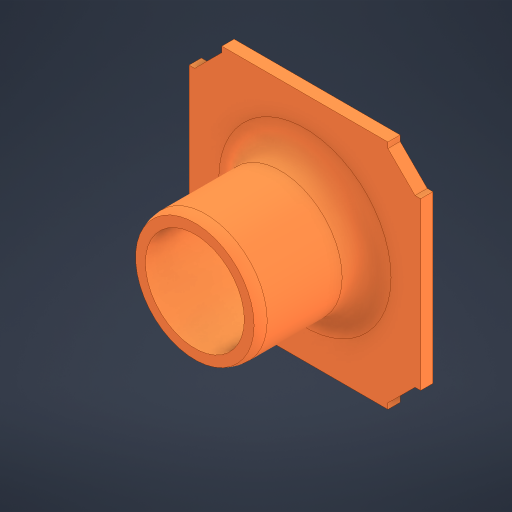
# Autodesk Inventor part: Objective Mount
Saved by Autodesk Inventor 2023.4 (Build 274418000, 418)
## iProperties
Created: 2022-08-09
Part Number: Objective Mount
Material: Generic
Document SubType Name: Modeling
Designer: xSibe
Density: 1 g/cm^3
Appearance: Plastic Orange
Author: xSibe
Autodesk Inventor part; units mm, degrees
ref_plane "YZ Plane" through (0, 0, 0) normal (1, 0, 0) x (0, 1, 0)
ref_plane "XZ Plane" through (0, 0, 0) normal (0, 1, 0) x (-1, 0, 0)
ref_plane "XY Plane" through (0, 0, 0) normal (0, 0, 1) x (1, 0, 0)
sketch "Sketch1" plane through (0, 0, 0) normal (0, 0, 1) x (1, 0, 0)
  circle A0 centre (-10, 20.9) radius 1.875 projected
  circle A1 centre (-10, -20.9) radius 1.875 projected
  circle A2 centre (10, 20.9) radius 1.875 projected
  circle A3 centre (10, -20.9) radius 1.875 projected
  circle A4 centre (20.8, -14.4) radius 2.075 projected
  circle A5 centre (20.8, 14.4) radius 2.075 projected
  circle A6 centre (-20.8, 14.4) radius 2.075 projected
  circle A7 centre (-20.8, -14.4) radius 2.075 projected
  line L0 (16.9, -16.9) -> (-16.9, -16.9) projected
  line L1 (-16.9, -16.9) -> (-16.9, 16.9) projected
  line L2 (-16.9, 16.9) -> (16.9, 16.9) projected
  line L3 (16.9, 16.9) -> (16.9, -16.9) projected
  line L4 (-17.05, 24.9) -> (-17.05, 22.55) projected
  line L5 (-17.05, 22.55) -> (-22.55, 17.05) projected
  line L6 (-22.55, 17.05) -> (-24.9, 17.05) projected
  line L7 (-24.9, 17.05) -> (-24.9, -17.05) projected
  line L8 (-24.9, -17.05) -> (-22.55, -17.05) projected
  line L9 (-22.55, -17.05) -> (-17.05, -22.55) projected
  line L10 (-17.05, -22.55) -> (-17.05, -24.9) projected
  line L11 (-17.05, -24.9) -> (17.05, -24.9) projected
  line L12 (17.05, -24.9) -> (17.05, -22.55) projected
  line L13 (17.05, -22.55) -> (22.55, -17.05) projected
  line L14 (22.55, -17.05) -> (24.9, -17.05) projected
  line L15 (24.9, -17.05) -> (24.9, 17.05) projected
  line L16 (24.9, 17.05) -> (22.55, 17.05) projected
  line L17 (22.55, 17.05) -> (17.05, 22.55) projected
  line L18 (17.05, 22.55) -> (17.05, 24.9) projected
  line L19 (17.05, 24.9) -> (-17.05, 24.9) projected
  line L20 (24.825, 16.975) -> (24.825, -16.975)
  line L21 (24.825, -16.975) -> (22.5189, -16.975)
  line L22 (22.5189, -16.975) -> (16.975, -22.5189)
  line L23 (16.975, -22.5189) -> (16.975, -24.825)
  line L24 (16.975, -24.825) -> (-16.975, -24.825)
  line L25 (-16.975, -24.825) -> (-16.975, -22.5189)
  line L26 (-16.975, -22.5189) -> (-22.5189, -16.975)
  line L27 (-22.5189, -16.975) -> (-24.825, -16.975)
  line L28 (-24.825, -16.975) -> (-24.825, 16.975)
  line L29 (-24.825, 16.975) -> (-22.5189, 16.975)
  line L30 (-22.5189, 16.975) -> (-16.975, 22.5189)
  line L31 (-16.975, 22.5189) -> (-16.975, 24.825)
  line L32 (-16.975, 24.825) -> (16.975, 24.825)
  line L33 (16.975, 24.825) -> (16.975, 22.5189)
  line L34 (16.975, 22.5189) -> (22.5189, 16.975)
  line L35 (22.5189, 16.975) -> (24.825, 16.975)
  line L36 (-24.825, 16.975) -> (-23.672, 16.975)
  line L37 (-23.672, 16.975) -> (-23.672, -16.975)
  line L38 (-23.672, -16.975) -> (-24.825, -16.975)
  line L39 (-24.825, -16.975) -> (-24.825, 16.975)
  line L40 (-16.975, 24.825) -> (16.975, 24.825)
  line L41 (16.975, 24.825) -> (16.975, 23.672)
  line L42 (16.975, 23.672) -> (-16.975, 23.672)
  line L43 (-16.975, 23.672) -> (-16.975, 24.825)
  line L44 (24.825, 16.975) -> (23.672, 16.975)
  line L45 (23.672, 16.975) -> (23.672, -16.975)
  line L46 (23.672, -16.975) -> (24.825, -16.975)
  line L47 (24.825, -16.975) -> (24.825, 16.975)
  line L48 (-16.975, -24.825) -> (16.975, -24.825)
  line L49 (16.975, -24.825) -> (16.975, -23.672)
  line L50 (16.975, -23.672) -> (-16.975, -23.672)
  line L51 (-16.975, -23.672) -> (-16.975, -24.825)
  point P0 (0, 0)
  dimension "d0" = 0.075
  constraints: 64 end point, 8 parallel, 4 horizontal, 4 midpoint, 4 perpendicular, 15 other
  measures "d0" distance between parallel lines of L15 L20
ref_plane "Work Plane1" through (-24.9, -24.9, 7.7) normal (0, 0, 1) x (1, 0, 0)
extrude "Extrusion1" add sketch "Sketch1" along normal blind 2.5 from surface at 7.7 contours A0 | A1 | A2 | A3 | A4 | A5 | A6 | A7 | L0 L1 L2 L3 | L45 L21 L22 L23 L50 L25 L26 L27 L37 L29 L30 L31 L42 L33 L34 L35
sketch "Sketch2" plane through (0, 0, 0) normal (0, 0, 1) x (1, 0, 0)
  line L0 (22.5189, 16.975) -> (23.672, 16.975) projected
  line L1 (16.975, 22.5189) -> (22.5189, 16.975) projected
  line L2 (16.975, 23.672) -> (16.975, 22.5189) projected
  line L3 (-16.975, 22.5189) -> (-16.975, 23.672) projected
  line L4 (-22.5189, 16.975) -> (-16.975, 22.5189) projected
  line L5 (-23.672, 16.975) -> (-22.5189, 16.975) projected
  line L6 (-22.5189, -16.975) -> (-23.672, -16.975) projected
  line L7 (-16.975, -22.5189) -> (-22.5189, -16.975) projected
  line L8 (-16.975, -23.672) -> (-16.975, -22.5189) projected
  line L9 (16.975, -22.5189) -> (16.975, -23.672) projected
  line L10 (22.5189, -16.975) -> (16.975, -22.5189) projected
  line L11 (23.672, -16.975) -> (22.5189, -16.975) projected
  line L12 (24.825, -16.975) -> (24.825, -24.825)
  line L13 (24.825, -24.825) -> (16.975, -24.825)
  line L14 (24.825, -24.825) -> (14.825, -24.825)
  line L15 (14.825, -24.825) -> (14.825, -19.825)
  line L16 (19.825, -14.825) -> (24.825, -14.825)
  line L17 (24.825, -14.825) -> (24.825, -24.825)
  line L18 (19.825, -14.825) -> (14.825, -19.825)
  line L19 (24.825, 24.825) -> (24.825, 14.825)
  line L20 (14.825, 24.825) -> (24.825, 24.825)
  line L21 (14.825, 19.825) -> (14.825, 24.825)
  line L22 (14.825, 19.825) -> (19.825, 14.825)
  line L23 (24.825, 14.825) -> (19.825, 14.825)
  line L24 (-24.825, 24.825) -> (-14.825, 24.825)
  line L25 (-24.825, 14.825) -> (-24.825, 24.825)
  line L26 (-19.825, 14.825) -> (-24.825, 14.825)
  line L27 (-19.825, 14.825) -> (-14.825, 19.825)
  line L28 (-14.825, 24.825) -> (-14.825, 19.825)
  line L29 (-24.825, -24.825) -> (-24.825, -14.825)
  line L30 (-14.825, -24.825) -> (-24.825, -24.825)
  line L31 (-14.825, -19.825) -> (-14.825, -24.825)
  line L32 (-14.825, -19.825) -> (-19.825, -14.825)
  line L33 (-24.825, -14.825) -> (-19.825, -14.825)
  line L34 (-16.975, -24.825) -> (16.975, -24.825)
  line L35 (16.975, -24.825) -> (16.975, -22.5189)
  line L36 (16.975, -22.5189) -> (-16.975, -22.5189)
  line L37 (-16.975, -22.5189) -> (-16.975, -24.825)
  line L38 (16.975, 22.5189) -> (-16.975, 22.5189)
  line L39 (-16.975, 22.5189) -> (-16.975, 24.825)
  line L40 (-16.975, 24.825) -> (16.975, 24.825)
  line L41 (16.975, 24.825) -> (16.975, 22.5189)
  line L42 (-24.825, 16.975) -> (-22.5189, 16.975)
  line L43 (-22.5189, 16.975) -> (-22.5189, -16.975)
  line L44 (-22.5189, -16.975) -> (-24.825, -16.975)
  line L45 (-24.825, -16.975) -> (-24.825, 16.975)
  line L46 (22.5189, -16.975) -> (24.825, -16.975)
  line L47 (24.825, -16.975) -> (24.825, 16.975)
  line L48 (24.825, 16.975) -> (22.5189, 16.975)
  line L49 (22.5189, 16.975) -> (22.5189, -16.975)
  circle A0 centre (0, 0) radius 10.1125
  circle A1 centre (0, 0) radius 12.6125
  line L50 (23.672, 16.975) -> (23.672, -16.975) projected
  line L51 (-16.975, 23.672) -> (16.975, 23.672) projected
  line L52 (-23.672, -16.975) -> (-23.672, 16.975) projected
  line L53 (16.975, -23.672) -> (-16.975, -23.672) projected
  point P0 (14.825, -14.825)
  point P1 (22.5189, -14.825)
  point P2 (22.5189, 14.825)
  point P3 (14.825, 22.5189)
  point P4 (-14.825, 22.5189)
  point P5 (-22.5189, 14.825)
  point P6 (-22.5189, -14.825)
  point P7 (-14.825, -22.5189)
  point P8 (14.825, -22.5189)
  dimension "d3" = 10
  dimension "d4" = 10
  dimension "d5" = 5
  dimension "d6" = 5
  dimension "d9" = 360
  dimension "d15" = 20.225
  dimension "d16" = 2.5
  constraints: 76 end point, 10 parallel, 6 perpendicular, 5 horizontal, 2 centre point, 2 point on line, 1 coincident, 1 vertical, 41 other
  measures "d3" distance of point (14.825, -14.825) L16.end
  measures "d4" distance of L14.end point (14.825, -14.825)
  measures "d5" distance of L16.start point (14.825, -14.825)
  measures "d6" distance of L15.end point (14.825, -14.825)
  measures "d15" diameter of A0
  measures "d16" radial gap between concentric circles of A0 A1
extrude "Extrusion2" add sketch "Sketch2" along normal blind 22.5 from surface at 10.2 contours A1
extrude "Extrusion3" cut sketch "Sketch2" against normal up to surface (2.5 mm away) from surface at 10.2 contours A0
chamfer "Chamfer1" distance 0.5 angle 45 1 edges at (-12.6125, 0, 32.7)
fillet "Fillet1" radius 5 2 edges at (-12.6125, 0, 10.2) (-12.6125, 0, 32.2)
equation "\"d6\" = d5"
body "Solid1"
